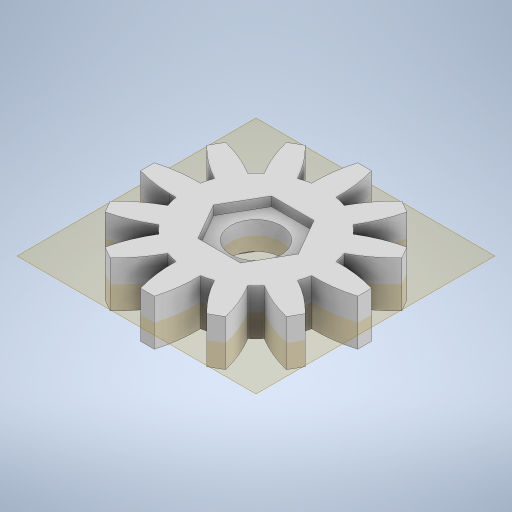
# Autodesk Inventor part: JointFixer
Saved by Autodesk Inventor 2023 (Build 270158000, 158)
## iProperties
Created: 2023-12-22
Part Number: JointFixer
Material: Generic
Document SubType Name: Modeling
Designer: Mustapha
Density: 1 g/cm^3
Appearance: Default
Author: Mustapha
Autodesk Inventor part; units mm, degrees
ref_plane "YZ Plane" through (0, 0, 0) normal (1, 0, 0) x (0, 1, 0)
ref_plane "XZ Plane" through (0, 0, 0) normal (0, 1, 0) x (-1, 0, 0)
ref_plane "XY Plane" through (0, 0, 0) normal (0, 0, 1) x (1, 0, 0)
sketch "Sketch1" plane through (0, 0, 0) normal (0, 1, 0) x (-1, 0, 0)
  circle A0 centre (0, 0) radius 7.5
  line L0 (8.0698, 1.3309) -> (7.381, 1.3309)
  line L1 (7.381, -1.3309) -> (8.0698, -1.3309)
  line L2 (12.3774, -0.5735) -> (12.3774, -0.474)
  line L3 (12.3774, 1.3309) -> (7.5, 0) construction
  line L4 (7.5, 0) -> (12.3774, -1.3309) construction
  line L5 (11.8209, 0) -> (11.8209, 0.7484)
  arc A1 (11.8209, 0.7484) -> (7.381, 1.3309) centre (7.7254, -13.2556) ccw
  line L6 (7.5, 0) -> (12.3774, 0)
  line L7 (12.3774, -1.3309) -> (7.5, 0) construction
  line L8 (11.8209, 0) -> (11.8209, -0.7484)
  arc A2 (7.381, -1.3309) -> (11.8209, -0.7484) centre (7.7254, 13.2556) ccw
  arc A3 (5.7266, -4.8431) -> (9.863, -6.5586) centre (13.3182, 7.617) ccw
  arc A4 (10.6114, -5.2623) -> (7.0576, -2.5379) centre (0.0626, -15.3424) ccw
  line L9 (10.2372, -5.9105) -> (10.6114, -5.2623)
  line L10 (10.2372, -5.9105) -> (9.863, -6.5586)
  arc A5 (2.5379, -7.0576) -> (5.2623, -10.6114) centre (15.3424, -0.0626) ccw
  arc A6 (6.5586, -9.863) -> (4.8431, -5.7266) centre (-7.617, -13.3182) ccw
  line L11 (5.9105, -10.2372) -> (6.5586, -9.863)
  line L12 (5.9105, -10.2372) -> (5.2623, -10.6114)
  arc A7 (-1.3309, -7.381) -> (-0.7484, -11.8209) centre (13.2556, -7.7254) ccw
  arc A8 (0.7484, -11.8209) -> (1.3309, -7.381) centre (-13.2556, -7.7254) ccw
  line L13 (0, -11.8209) -> (0.7484, -11.8209)
  line L14 (0, -11.8209) -> (-0.7484, -11.8209)
  arc A9 (-4.8431, -5.7266) -> (-6.5586, -9.863) centre (7.617, -13.3182) ccw
  arc A10 (-5.2623, -10.6114) -> (-2.5379, -7.0576) centre (-15.3424, -0.0626) ccw
  line L15 (-5.9105, -10.2372) -> (-5.2623, -10.6114)
  line L16 (-5.9105, -10.2372) -> (-6.5586, -9.863)
  arc A11 (-7.0576, -2.5379) -> (-10.6114, -5.2623) centre (-0.0626, -15.3424) ccw
  arc A12 (-9.863, -6.5586) -> (-5.7266, -4.8431) centre (-13.3182, 7.617) ccw
  line L17 (-10.2372, -5.9105) -> (-9.863, -6.5586)
  line L18 (-10.2372, -5.9105) -> (-10.6114, -5.2623)
  arc A13 (-7.381, 1.3309) -> (-11.8209, 0.7484) centre (-7.7254, -13.2556) ccw
  arc A14 (-11.8209, -0.7484) -> (-7.381, -1.3309) centre (-7.7254, 13.2556) ccw
  line L19 (-11.8209, 0) -> (-11.8209, -0.7484)
  line L20 (-11.8209, 0) -> (-11.8209, 0.7484)
  arc A15 (-5.7266, 4.8431) -> (-9.863, 6.5586) centre (-13.3182, -7.617) ccw
  arc A16 (-10.6114, 5.2623) -> (-7.0576, 2.5379) centre (-0.0626, 15.3424) ccw
  line L21 (-10.2372, 5.9105) -> (-10.6114, 5.2623)
  line L22 (-10.2372, 5.9105) -> (-9.863, 6.5586)
  arc A17 (-2.5379, 7.0576) -> (-5.2623, 10.6114) centre (-15.3424, 0.0626) ccw
  arc A18 (-6.5586, 9.863) -> (-4.8431, 5.7266) centre (7.617, 13.3182) ccw
  line L23 (-5.9105, 10.2372) -> (-6.5586, 9.863)
  line L24 (-5.9105, 10.2372) -> (-5.2623, 10.6114)
  arc A19 (1.3309, 7.381) -> (0.7484, 11.8209) centre (-13.2556, 7.7254) ccw
  arc A20 (-0.7484, 11.8209) -> (-1.3309, 7.381) centre (13.2556, 7.7254) ccw
  line L25 (0, 11.8209) -> (-0.7484, 11.8209)
  line L26 (0, 11.8209) -> (0.7484, 11.8209)
  arc A21 (4.8431, 5.7266) -> (6.5586, 9.863) centre (-7.617, 13.3182) ccw
  arc A22 (5.2623, 10.6114) -> (2.5379, 7.0576) centre (15.3424, 0.0626) ccw
  line L27 (5.9105, 10.2372) -> (5.2623, 10.6114)
  line L28 (5.9105, 10.2372) -> (6.5586, 9.863)
  arc A23 (7.0576, 2.5379) -> (10.6114, 5.2623) centre (0.0626, 15.3424) ccw
  arc A24 (9.863, 6.5586) -> (5.7266, 4.8431) centre (13.3182, -7.617) ccw
  line L29 (10.2372, 5.9105) -> (9.863, 6.5586)
  line L30 (10.2372, 5.9105) -> (10.6114, 5.2623)
  line L31 (2.6226, -0.9781) -> (2.6226, -1.001)
  line L32 (2.6226, 1.001) -> (2.6226, 0.9781)
  line L33 (2.6226, 0.4136) -> (2.6226, 0.391)
  circle A25 centre (0, 0) radius 2.75
  point P0 (10.4324, -6.6853)
  point P1 (6.3232, -5.1875)
  point P2 (7.6541, -2.8823)
  point P3 (5.692, -11.0058)
  point P4 (2.8823, -7.6541)
  point P5 (5.1875, -6.3232)
  point P6 (-0.5735, -12.3774)
  point P7 (-1.3309, -8.0698)
  point P8 (1.3309, -8.0698)
  point P9 (-6.6853, -10.4324)
  point P10 (-5.1875, -6.3232)
  point P11 (-2.8823, -7.6541)
  point P12 (-11.0058, -5.692)
  point P13 (-7.6541, -2.8823)
  point P14 (-6.3232, -5.1875)
  point P15 (-12.3774, 0.5735)
  point P16 (-8.0698, 1.3309)
  point P17 (-8.0698, -1.3309)
  point P18 (-10.4324, 6.6853)
  point P19 (-6.3232, 5.1875)
  point P20 (-7.6541, 2.8823)
  point P21 (-5.692, 11.0058)
  point P22 (-2.8823, 7.6541)
  point P23 (-5.1875, 6.3232)
  point P24 (0.5735, 12.3774)
  point P25 (1.3309, 8.0698)
  point P26 (-1.3309, 8.0698)
  point P27 (6.6853, 10.4324)
  point P28 (5.1875, 6.3232)
  point P29 (2.8823, 7.6541)
  point P30 (11.0058, 5.692)
  point P31 (7.6541, 2.8823)
  point P32 (6.3232, 5.1875)
  point P33 (7.0576, -2.5379)
  point P34 (7.0576, 2.5379)
  point P35 (5.7266, 4.8431)
  point P36 (4.8431, 5.7266)
  point P37 (2.5379, 7.0576)
  point P38 (1.3309, 7.381)
  point P39 (-1.3309, 7.381)
  point P40 (-2.5379, 7.0576)
  point P41 (-4.8431, 5.7266)
  point P42 (-5.7266, 4.8431)
  point P43 (-7.0576, 2.5379)
  point P44 (-7.381, 1.3309)
  point P45 (-7.381, -1.3309)
  point P46 (-7.0576, -2.5379)
  point P47 (-5.7266, -4.8431)
  point P48 (-4.8431, -5.7266)
  point P49 (-2.5379, -7.0576)
  point P50 (-1.3309, -7.381)
  point P51 (1.3309, -7.381)
  point P52 (2.5379, -7.0576)
  point P53 (4.8431, -5.7266)
  dimension "d0" = 15
  dimension "d3" = 360
  dimension "d5" = 5.5
  constraints: 91 point on circle, 70 end point, 25 centre point, 4 parallel, 3 perpendicular, 3 symmetric about line, 2 coincident, 1 horizontal, 1 vertical, 174 other
  measures "d5" diameter of A25
extrude "Extrusion1" add sketch "Sketch1" along normal blind 5 contours A0 | L6 L8 A2 L1 A0 | A0 L0 A1 L5 L6 | A0 A24 L29 L30 A23 | A4 L9 L10 A3 A0 | A0 A22 L27 L28 A21 | A6 L11 L12 A5 A0 | A0 A20 L25 L26 A19 | A8 L13 L14 A7 A0 | A0 A18 L23 L24 A17 | A10 L15 L16 A9 A0 | A0 A16 L21 L22 A15 | A12 L17 L18 A11 A0 | A0 A14 L19 L20 A13
sketch "Sketch2" plane through (0, 5, 0) normal (0, 1, 0) x (1, 0, 0)
  line L0 (-2.3094, 4) -> (2.3094, 4)
  line L1 (2.3094, 4) -> (4.6188, 0)
  line L2 (4.6188, 0) -> (2.3094, -4)
  line L3 (2.3094, -4) -> (-2.3094, -4)
  line L4 (-2.3094, -4) -> (-4.6188, 0)
  line L5 (-4.6188, 0) -> (-2.3094, 4)
  line L6 (0, 0) -> (-6.3613, 0)
  dimension "d8" = 8
  constraints: 14 end point, 1 coincident, 1 horizontal, 1 parallel, 13 other
  measures "d8" distance between parallel lines of L3 L0
extrude "Extrusion2" cut sketch "Sketch2" against normal blind 1
ref_plane "Work Plane1" through (0, 2.5, 0) normal (0, 1, 0) x (1, 0, 0)
mirror "Mirror1" about plane through (0, 2.5, 0) normal (0, 1, 0) of "Extrusion2"
body "Solid1"
